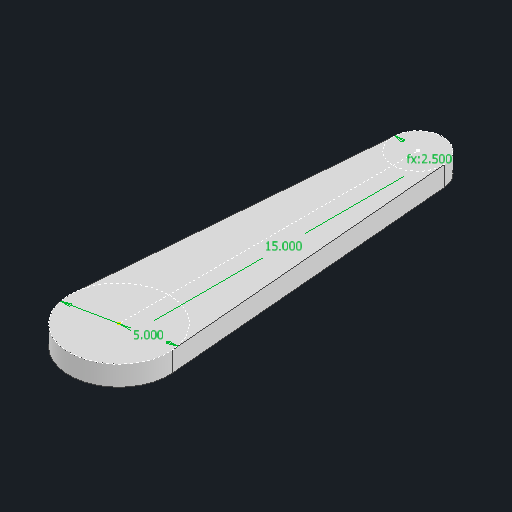
# Autodesk Inventor part: Post
Saved by Autodesk Inventor 2023.1 (Build 271208000, 208)
## iProperties
Created: 2022-12-06
Part Number: Post
Material: Generic
Document SubType Name: Modeling
Designer: aubrey-work
Density: 1 g/cm^3
Appearance: Default
majorDiameter: 5.000 in
armLength: 15.000 in
minorDiameter: 2.500 in
armThickness: 1.000 in
d4: 0.00 deg
Author: aubrey-work
Autodesk Inventor part; units mm, degrees
ref_plane "YZ Plane" through (0, 0, 0) normal (1, 0, 0) x (0, 1, 0)
ref_plane "XZ Plane" through (0, 0, 0) normal (0, 1, 0) x (-1, 0, 0)
ref_plane "XY Plane" through (0, 0, 0) normal (0, 0, 1) x (1, 0, 0)
sketch "Sketch1" plane through (0, 0, 0) normal (0, 1, 0) x (-1, 0, 0)
  circle A0 centre (0, 0) radius 63.5 construction
  line L0 (0, 0) -> (0, -381) construction
  circle A1 centre (0, -381) radius 31.75 construction
  dimension "majorDiameter" = 127
  dimension "armLength" = 381
  dimension "minorDiameter" = 63.5
  constraints: 2 centre point, 2 coincident, 2 end point, 1 vertical
  measures "majorDiameter" diameter of A0
  measures "armLength" distance of L0.start L0.end
  measures "minorDiameter" diameter of A1
sketch "Sketch2" plane through (0, 0, 0) normal (0, 1, 0) x (-1, 0, 0)
  line L0 (63.2791, -5.2917) -> (31.6396, -383.6458)
  line L1 (-31.6396, -383.6458) -> (-63.2791, -5.2917)
  circle A0 centre (0, -381) radius 31.75 construction
  circle A1 centre (0, 0) radius 63.5 construction
  arc A2 (-31.6396, -383.6458) -> (31.6396, -383.6458) centre (0, -381) ccw
  arc A3 (63.2791, -5.2917) -> (-63.2791, -5.2917) centre (0, 0) ccw
  constraints: 8 point on circle, 6 tangent, 4 end point, 2 centre point
extrude "Extrusion1" add sketch "Sketch2" against normal blind 25.4
equation "\"minorDiameter\" = 0.5 * majorDiameter"
body "Solid1"
